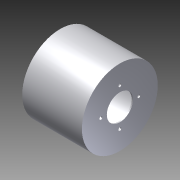
# Autodesk Inventor part: rim_8 in x 6.3 in
Saved by Autodesk Inventor 2012 (Build 160160000, 160)
## iProperties
Created: 2011-11-26
Part Number: rim_8 in x 6.3 in
Material: Default
Document SubType Name: Modeling
Designer: Antonella
Density: 1 g/cm^3
Mass: 1631.03 g
Surface Area: 2363.67 cm^2
Volume: 1631.03 cm^3
Author: Antonella
Autodesk Inventor part; units mm, degrees
ref_plane "YZ Plane" through (0, 0, 0) normal (1, 0, 0) x (0, 1, 0)
ref_plane "XZ Plane" through (0, 0, 0) normal (0, 1, 0) x (-1, 0, 0)
ref_plane "XY Plane" through (0, 0, 0) normal (0, 0, 1) x (1, 0, 0)
sketch "Sketch1" plane through (0, 0, 0) normal (0, 0, 1) x (1, 0, 0)
  line L0 (-179.5854, 0) -> (123.2759, 0) projected
  line L1 (0, -20.32) -> (0, 121.92) projected
  line L2 (-80.01, 101.6) -> (80.01, 101.6)
  line L3 (80.01, 50.8) -> (-80.01, 50.8) construction
  line L4 (80.01, 0) -> (-136.3195, 0) construction
  arc A0 (-80.01, 101.6) -> (-76.835, 98.425) centre (-76.835, 101.6) ccw
  line L5 (60.96, 85.725) -> (-64.135, 85.725)
  arc A1 (-76.835, 98.425) -> (-64.135, 85.725) centre (-64.135, 98.425) ccw
  arc A2 (67.31, 66.675) -> (76.835, 57.15) centre (76.835, 66.675) ccw
  arc A3 (67.31, 79.375) -> (60.96, 85.725) centre (60.96, 79.375) ccw
  line L6 (67.31, 79.375) -> (67.31, 66.675)
  line L7 (80.01, 101.6) -> (80.01, 0)
  line L8 (80.01, 98.425) -> (-76.835, 98.425) construction
  line L9 (-64.135, 85.725) -> (-64.135, 101.6) construction
  line L10 (-76.835, 98.425) -> (-76.835, 101.6) construction
  line L11 (60.96, 85.725) -> (80.01, 85.725) construction
  line L12 (67.31, 79.375) -> (80.01, 79.375) construction
  line L13 (60.96, 50.8) -> (60.96, 101.6) construction
  line L14 (67.31, 66.675) -> (80.01, 66.675) construction
  line L15 (76.835, 57.15) -> (76.835, 0)
  line L16 (76.835, 57.15) -> (80.01, 57.15) construction
  line L17 (76.835, 0) -> (80.01, 0)
  point P0 (0, 0)
  point P1 (0, 101.6)
  dimension "d0" = 101.6
  dimension "d2" = 160.02
  dimension "d4" = 50.8
  dimension "d10" = 6.35
  dimension "d11" = 12.7
  dimension "d13" = 3.175
  dimension "d14" = 34.925
  dimension "d15" = 19.05
  dimension "d16" = 12.7
  constraints: 32 end point, 13 point on line, 8 point on circle, 8 tangent, 7 perpendicular, 4 centre point, 3 parallel, 2 collinear, 2 midpoint, 1 horizontal alignment, 1 vertical alignment
  measures "d0" distance between parallel lines of L2 L0
  measures "d2" distance of L2.start L2.end
  measures "d4" distance between parallel lines of L3 L0
  measures "d10" radius of A3
  measures "d11" distance between parallel lines of L8 L5
  measures "d13" distance between parallel lines of L7 L15
  measures "d14" distance between parallel lines of L11 L3
  measures "d15" distance between parallel lines of L7 L13
  measures "d16" distance between parallel lines of L12 L14
revolve "Revolution1" add sketch "Sketch1" angle 360 about axis through (-10, 0, 0) along (1, 0, 0) contours L15 A2 L6 A3 L5 L1 L2 L7 L0 | L5 A1 A0 L2 L1
sketch "Sketch2" plane through (76.835, 0, 0) normal (-1, 0, 0) x (0, 0, 1)
  circle A0 centre (0, 0) radius 57.15 projected
  circle A1 centre (0, 0) radius 50.8 construction
  circle A2 centre (0, 0) radius 34.925
  circle A3 centre (0, 50.8) radius 4.0132
  circle A4 centre (-50.8, 0) radius 4.0132
  circle A5 centre (0, -50.8) radius 4.0132
  circle A6 centre (50.8, 0) radius 4.0132
  dimension "d18" = 101.6
  dimension "d19" = 69.85
  dimension "d20" = 8.0264
  dimension "d23" = 360
  constraints: 5 centre point, 2 coincident, 2 vertical alignment, 11 other
  measures "d19" diameter of A2
  measures "d20" diameter of A3
extrude "Extrusion1" cut sketch "Sketch2" against normal through all contours A2 | A3 | A4 | A5 | A6
body "Solid1"
